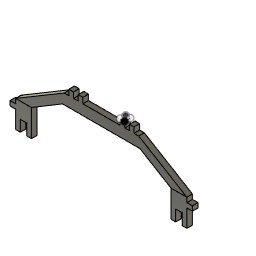
Test frame parts v2 (Autodesk Fusion 360 archive; units mm, degrees)
design "Test Carry Legs"
Autodesk Fusion 360 part; units mm, degrees
sketch "Sketch1" plane through (0, 0, 0) normal (0, 0, 1) x (1, 0, 0) in component "sidelegs"
  line L0 (-75, -45) -> (-92, -45)
  line L1 (-92, -45) -> (-92, -39)
  line L2 (-92, -39) -> (-75, -39)
  line L3 (-75, -39) -> (-75, -45)
  line L4 (75, -45) -> (92, -45)
  line L5 (92, -45) -> (92, -39)
  line L6 (92, -39) -> (75, -39)
  line L7 (75, -39) -> (75, -45)
  dimension "d7" = 17
  dimension "d8" = 6
  dimension "d9" = 17
  dimension "d10" = 6
  constraint horizontal L0
  constraint vertical L1
  constraint horizontal L2
  constraint vertical L3
  constraint horizontal L4
  constraint vertical L5
  constraint horizontal L6
  constraint vertical L7
  measures "d7" distance of L0.start L0.end
  measures "d8" distance of L0.start L2.end
  measures "d9" distance of L4.start L4.end
  measures "d10" distance of L4.start L6.end
extrude "Extrude1" add sketch "Sketch1" along normal blind 17 makes body 1 at (-80.6667, -45, 11.3333) makes body 2 at (86.3333, -39, 11.3333) in component "sidelegs"
sketch "Sketch2" plane through (0, -45, 0) normal (0, -1, 0) x (1, 0, 0) in component "sidelegs"
  line L0 (-92, 0) -> (-75, 0)
  line L1 (-75, 0) -> (-75, 17)
  line L2 (-75, 17) -> (-92, 17)
  line L3 (-92, 17) -> (-92, 0)
  line L4 (-75, 17) -> (-41.5705, 37.0865)
  line L5 (-75, 17) -> (-36, 17) construction
  line L6 (75, 17) -> (41.5705, 37.0865)
  line L7 (75, 17) -> (114, 17) construction
  line L8 (-41.5705, 37.0865) -> (41.5705, 37.0865)
  line L9 (92, 17) -> (40.2293, 48.107)
  line L10 (40.2293, 48.107) -> (-39.7707, 48.107)
  line L11 (-39.7707, 48.107) -> (-92, 17)
  line L12 (75, 17) -> (92, 17)
  line L13 (-75, 17) -> (-92, 17)
  dimension "d13" = 39
  dimension "d14" = 31
  dimension "d15" = 149
  dimension "d16" = 39
  dimension "d25" = 80
  constraint horizontal L5
  constraint coincident L1.end L2.start
  constraint horizontal L7
  constraint coincident L7 L9.start
  constraint parallel L6 L9
  constraint parallel L7 L10
  constraint coincident L2.end L3.start
  measures "d13" distance of L1.end L4.end
  measures "d14" angle of L4 L5
  measures "d15" angle of L6 L7
  measures "d16" distance of L6.start L6.end
  measures "d25" distance of L9.end L10.end
extrude "Extrude2" add sketch "Sketch2" against normal blind 6 separate body contours L2 L4 L6 L8 L9 L10 L11 L12 L13 makes body 3 in component "sidelegs"
sketch "Sketch3" plane through (0, 0, 0) normal (0, 0, -1) x (1, 0, 0) in component "sidelegs"
  line L0 (-92, 39) -> (-75, 39)
  line L1 (-75, 39) -> (-75, 45)
  line L2 (-75, 45) -> (-92, 45)
  line L3 (-92, 45) -> (-92, 39)
  line L4 (-92, 45) -> (-87, 45)
  line L5 (-87, 45) -> (-87, 39)
  line L6 (-87, 39) -> (-92, 39)
  line L7 (-92, 39) -> (-92, 45)
  line L8 (-75, 45) -> (-80, 45)
  line L9 (-80, 45) -> (-80, 39)
  line L10 (-80, 39) -> (-75, 39)
  line L11 (-75, 39) -> (-75, 45)
  constraint horizontal L4
  constraint vertical L5
  constraint horizontal L6
  constraint vertical L7
  constraint coincident L0 L5.end
  constraint coincident L2.end L3.start
  constraint horizontal L8
  constraint vertical L9
  constraint horizontal L10
  constraint vertical L11
  constraint coincident L0 L9.end
  constraint coincident L1.end L2.start
extrude "Extrude3" add sketch "Sketch3" along normal blind 12 contours L0 L2 L3 L4 L5 L6 L7 | L0 L1 L2 L8 L9 L10 L11 bodies 1 in component "sidelegs"
ref_plane "WorkPlane1" through (0, 0, 0) normal (1, 0, 0) x (0, 1, 0) in component "sidelegs"
sketch "Sketch4" plane through (0, 0, 0) normal (0, 0, -1) x (1, 0, 0) in component "sidelegs"
  line L0 (75, 45) -> (75, 39)
  line L1 (75, 39) -> (92, 39)
  line L2 (92, 39) -> (92, 45)
  line L3 (92, 45) -> (75, 45)
  line L4 (92, 39) -> (87, 39)
  line L5 (87, 39) -> (87, 45)
  line L6 (87, 45) -> (92, 45)
  line L7 (92, 45) -> (92, 39)
  line L8 (75, 39) -> (80, 39)
  line L9 (80, 39) -> (80, 45)
  line L10 (80, 45) -> (75, 45)
  line L11 (75, 45) -> (75, 39)
  constraint horizontal L4
  constraint vertical L5
  constraint horizontal L6
  constraint vertical L7
  constraint coincident L3 L5.end
  constraint coincident L1.end L2.start
  constraint horizontal L8
  constraint vertical L9
  constraint horizontal L10
  constraint vertical L11
  constraint coincident L3 L9.end
  constraint coincident L0.end L1.start
extrude "Extrude4" add sketch "Sketch4" along normal blind 12 contours L0 L1 L3 L8 L9 L10 L11 | L1 L2 L3 L4 L5 L6 L7 bodies 2 in component "sidelegs"
sketch "Sketch5" plane through (0, 0, 48.107) normal (0, 0, 1) x (-1, 0, 0) in component "sidelegs"
  line L0 (39.7707, 45) -> (-40.2293, 45)
  line L1 (-40.2293, 45) -> (-40.2293, 39)
  line L2 (-40.2293, 39) -> (39.7707, 39)
  line L3 (39.7707, 39) -> (39.7707, 45)
  line L4 (-40.2293, 45) -> (-35.2293, 45) construction
  line L5 (-35.2293, 45) -> (-35.2293, 39) construction
  line L6 (-35.2293, 39) -> (-40.2293, 39) construction
  line L7 (-40.2293, 39) -> (-40.2293, 45) construction
  line L8 (39.7707, 45) -> (34.7707, 45) construction
  line L9 (34.7707, 45) -> (34.7707, 39) construction
  line L10 (34.7707, 39) -> (39.7707, 39) construction
  line L11 (39.7707, 39) -> (39.7707, 45) construction
  line L12 (-35.2293, 45) -> (-30.2293, 45) construction
  line L13 (-30.2293, 45) -> (-30.2293, 39) construction
  line L14 (-30.2293, 39) -> (-35.2293, 39) construction
  line L15 (-35.2293, 39) -> (-35.2293, 45) construction
  line L16 (-30, 45) -> (-25, 45) construction
  line L17 (-25, 45) -> (-25, 39) construction
  line L18 (-25, 39) -> (-30, 39) construction
  line L19 (-30, 39) -> (-30, 45) construction
  line L20 (34.7707, 45) -> (29.7707, 45) construction
  line L21 (29.7707, 45) -> (29.7707, 39) construction
  line L22 (29.7707, 39) -> (34.7707, 39) construction
  line L23 (34.7707, 39) -> (34.7707, 45) construction
  line L24 (29.7707, 45) -> (24.7707, 45) construction
  line L25 (24.7707, 45) -> (24.7707, 39) construction
  line L26 (24.7707, 39) -> (29.7707, 39) construction
  line L27 (29.7707, 39) -> (29.7707, 45) construction
  line L28 (34.7707, 45) -> (29.7707, 45)
  line L29 (29.7707, 45) -> (29.7707, 39)
  line L30 (29.7707, 39) -> (34.7707, 39)
  line L31 (34.7707, 39) -> (34.7707, 45)
  line L32 (-35.2293, 45) -> (-30, 45)
  line L33 (-30, 45) -> (-30, 39)
  line L34 (-30, 39) -> (-35.2293, 39)
  line L35 (-35.2293, 39) -> (-35.2293, 45)
  line L36 (-25, 45) -> (-20, 45)
  line L37 (-20, 45) -> (-20, 39)
  line L38 (-20, 39) -> (-25, 39)
  line L39 (-25, 39) -> (-25, 45)
  line L40 (24.7707, 45) -> (19.7707, 45)
  line L41 (19.7707, 45) -> (19.7707, 39)
  line L42 (19.7707, 39) -> (24.7707, 39)
  line L43 (24.7707, 39) -> (24.7707, 45)
  dimension "d26" = 5
  dimension "d27" = 5
  dimension "d28" = 5
  dimension "d29" = 5
  dimension "d30" = 5
  dimension "d31" = 5
  dimension "d32" = 5
  constraint horizontal L4
  constraint vertical L5
  constraint horizontal L6
  constraint vertical L7
  constraint coincident L2 L5.end
  constraint coincident L0.end L1.start
  constraint horizontal L8
  constraint vertical L9
  constraint horizontal L10
  constraint vertical L11
  constraint coincident L2 L9.end
  constraint coincident L0.start L3.end
  constraint horizontal L12
  constraint vertical L13
  constraint horizontal L14
  constraint vertical L15
  constraint coincident L2 L13.end
  constraint horizontal L16
  constraint vertical L17
  constraint horizontal L18
  constraint vertical L19
  constraint coincident L0 L16.start
  constraint horizontal L20
  constraint vertical L21
  constraint horizontal L22
  constraint vertical L23
  constraint coincident L2 L21.end
  constraint horizontal L24
  constraint vertical L25
  constraint horizontal L26
  constraint vertical L27
  constraint coincident L2 L25.end
  constraint horizontal L28
  constraint vertical L29
  constraint horizontal L30
  constraint vertical L31
  constraint horizontal L32
  constraint vertical L33
  constraint horizontal L34
  constraint vertical L35
  constraint horizontal L36
  constraint vertical L37
  constraint horizontal L38
  constraint vertical L39
  constraint coincident L2 L37.end
  constraint horizontal L40
  constraint vertical L41
  constraint horizontal L42
  constraint vertical L43
  measures "d26" distance of L0.end L4.end
  measures "d27" distance of L0.start L8.end
  measures "d28" distance of L4.end L12.end
  measures "d29" distance of L16.start L16.end
  measures "d30" distance of L8.end L20.end
  measures "d31" distance of L20.end L24.end
  measures "d32" distance of L24.end L40.end
extrude "Extrude5" add sketch "Sketch5" along normal blind 6 contours L0 L2 L28 L29 L30 L31 | L0 L2 L40 L41 L42 L43 | L0 L2 L36 L37 L38 L39 | L0 L2 L32 L33 L34 L35 bodies 3 in component "sidelegs"
sketch "Sketch6" plane through (-92, 0, 0) normal (-1, 0, 0) x (0, -1, 0) in component "sidelegs"
  line L0 (45, -12) -> (45, 17)
  line L1 (45, 17) -> (39, 17)
  line L2 (39, 17) -> (39, -12)
  line L3 (39, -12) -> (45, -12)
  line L4 (45, 17) -> (45, 0) construction
  line L5 (39, 0) -> (39, 17) construction
  line L6 (39, 17) -> (45, 17) construction
  line L7 (45, 17) -> (45, 12) construction
  line L8 (45, 12) -> (39, 12) construction
  line L9 (39, 12) -> (39, 17) construction
  line L10 (39, 12) -> (45, 12)
  line L11 (45, 12) -> (45, 7)
  line L12 (45, 7) -> (39, 7)
  line L13 (39, 7) -> (39, 12)
  constraint coincident L0.end L1.start
  constraint coincident L0 L4.end
  constraint perpendicular L1 L4
  constraint coincident L2 L5.start
  constraint coincident L1.end L2.start
  constraint horizontal L6
  constraint vertical L7
  constraint horizontal L8
  constraint vertical L9
  constraint coincident L4 L7.end
  constraint horizontal L10
  constraint vertical L11
  constraint horizontal L12
  constraint vertical L13
  constraint coincident L4 L11.end
extrude "Extrude6" add sketch "Sketch6" along normal blind 6 contours L0 L2 L10 L11 L12 L13 bodies 1 in component "sidelegs"
sketch "Sketch7" plane through (92, 0, 0) normal (1, 0, 0) x (0, 1, 0) in component "sidelegs"
  line L0 (-39, -12) -> (-39, 17)
  line L1 (-39, 17) -> (-45, 17)
  line L2 (-45, 17) -> (-45, -12)
  line L3 (-45, -12) -> (-39, -12)
  line L4 (-45, 17) -> (-39, 17) construction
  line L5 (-39, 17) -> (-39, 12) construction
  line L6 (-39, 12) -> (-45, 12) construction
  line L7 (-45, 12) -> (-45, 17) construction
  line L8 (-45, 12) -> (-39, 12)
  line L9 (-39, 12) -> (-39, 7)
  line L10 (-39, 7) -> (-45, 7)
  line L11 (-45, 7) -> (-45, 12)
  constraint horizontal L4
  constraint vertical L5
  constraint horizontal L6
  constraint vertical L7
  constraint coincident L0 L5.end
  constraint coincident L1.end L2.start
  constraint horizontal L8
  constraint vertical L9
  constraint horizontal L10
  constraint vertical L11
  constraint coincident L0 L9.end
extrude "Extrude7" add sketch "Sketch7" along normal blind 6 contours L0 L2 L8 L9 L10 L11 bodies 2 in component "sidelegs"
sketch "Sketch8" plane through (0, 0, 54.107) normal (0, 0, 1) x (-1, 0, 0) in component "sidelegs"
  line L0 (-35.2293, 39) -> (-30, 39)
  line L1 (-30, 39) -> (-30, 45)
  line L2 (-30, 45) -> (-35.2293, 45)
  line L3 (-35.2293, 45) -> (-35.2293, 39)
  line L4 (-30, 42) -> (-30.229, 42) construction
  line L5 (-30.229, 42) -> (-30.229, 39) construction
  line L6 (-30.229, 42) -> (-30.229, 45) construction
  line L7 (-30.229, 45) -> (-30, 45) construction
  line L8 (-30, 45) -> (-30, 39) construction
  line L9 (-30, 39) -> (-30.229, 39) construction
  line L10 (-30.229, 39) -> (-30.229, 45) construction
  line L11 (-30, 45) -> (-30.229, 45)
  line L12 (-30.229, 45) -> (-30.229, 39)
  line L13 (-30.229, 39) -> (-30, 39)
  line L14 (-30, 39) -> (-30, 45)
  dimension "d39" = 0.229
  constraint midpoint L1 L4.start
  constraint perpendicular L1 L4
  constraint coincident L0 L5.end
  constraint perpendicular L0 L5
  constraint coincident L2 L6.end
  constraint perpendicular L2 L6
  constraint horizontal L7
  constraint vertical L8
  constraint horizontal L9
  constraint vertical L10
  constraint coincident L0.end L1.start
  constraint horizontal L11
  constraint vertical L12
  constraint horizontal L13
  constraint vertical L14
  measures "d39" distance of L4.start L4.end
extrude "Extrude8" cut sketch "Sketch8" against normal blind 6 contours L0 L1 L2 L11 L12 L13 L14 bodies 3 in component "sidelegs"
sketch "Sketch9" plane through (0, 0, 54.107) normal (0, 0, 1) x (-1, 0, 0) in component "sidelegs"
  line L0 (-25, 39) -> (-20, 39)
  line L1 (-20, 39) -> (-20, 45)
  line L2 (-20, 45) -> (-25, 45)
  line L3 (-25, 45) -> (-25, 39)
  line L4 (-25, 45) -> (-25.229, 45)
  line L5 (-25.229, 45) -> (-25.229, 39)
  line L6 (-25.229, 39) -> (-25, 39)
  line L7 (-20.229, 45) -> (-20.229, 39)
  dimension "d42" = 0.229
  dimension "d43" = 6
  dimension "d46" = 0.229
  constraint horizontal L4
  constraint vertical L5
  constraint horizontal L6
  constraint coincident L2.end L3.start
  constraint vertical L7
  constraint coincident L0 L7.end
  measures "d42" distance of L2.end L4.end
  measures "d43" distance of L2.end L0.start
  measures "d46" distance of L1.end L7.start
extrude "Extrude9" add sketch "Sketch9" against normal blind 6 contours L3 L4 L5 L6 bodies 3 in component "sidelegs"
extrude "Extrude10" cut sketch "Sketch9" against normal blind 6 contours L0 L1 L2 L7 bodies 3 in component "sidelegs"
component "sidelegs" placed x (1, 0, 0) y (0, 1, 0) z (0, 0, 1) at (0, 0, 0)

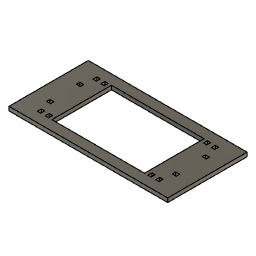
design "Test Base"
Autodesk Fusion 360 part; units mm, degrees
sketch "Sketch1" plane through (0, 0, 0) normal (0, 0, 1) x (1, 0, 0) in component "Base"
  line L0 (120, 60) -> (-120, 60)
  line L1 (-120, 60) -> (-120, -60)
  line L2 (-120, -60) -> (120, -60)
  line L3 (120, -60) -> (120, 60)
  line L4 (120, 60) -> (-120, -60) construction
  line L5 (-120, 60) -> (120, -60) construction
  line L6 (-70, 45) -> (70, 45)
  line L7 (70, 45) -> (70, -45)
  line L8 (70, -45) -> (-70, -45)
  line L9 (-70, -45) -> (-70, 45)
  line L10 (-70, 45) -> (70, -45) construction
  line L11 (70, 45) -> (-70, -45) construction
  dimension "d1" = 240
  dimension "d2" = 120
  dimension "d3" = 90
  dimension "d6" = 140
  constraint horizontal L0
  constraint perpendicular L0 L1
  constraint parallel L0 L2
  constraint parallel L1 L3
  constraint coincident L4 origin
  constraint coincident L5 origin
  constraint horizontal L6
  constraint perpendicular L6 L7
  constraint parallel L6 L8
  constraint parallel L7 L9
  constraint coincident L10 origin
  constraint coincident L11 origin
  measures "d1" distance of L1.end L2.end
  measures "d2" distance of L0.end L1.end
  measures "d3" distance of L6.end L7.end
  measures "d6" distance of L7 L9
extrude "Extrude1" add sketch "Sketch1" along normal blind 6 in component "Base"
sketch "Sketch2" plane through (0, 0, 6) normal (0, 0, 1) x (-1, 0, 0) in component "Base"
  line L0 (-70, 45) -> (70, 45)
  line L1 (70, 45) -> (70, -45)
  line L2 (70, -45) -> (-70, -45)
  line L3 (-70, -45) -> (-70, 45)
  line L4 (-120, 60) -> (-120, -60)
  line L5 (-120, -60) -> (120, -60)
  line L6 (120, -60) -> (120, 60)
  line L7 (120, 60) -> (-120, 60)
  line L8 (70, 45) -> (92, 45) construction
  line L9 (92, 45) -> (92, 39) construction
  line L10 (92, 39) -> (70, 39) construction
  line L11 (70, 39) -> (70, 45) construction
  line L12 (92, 39) -> (87, 39)
  line L13 (87, 39) -> (87, 45)
  line L14 (87, 45) -> (92, 45)
  line L15 (92, 45) -> (92, 39)
  line L16 (70, 39) -> (75, 39) construction
  line L17 (75, 45) -> (75, 39) construction
  line L18 (75, 39) -> (80, 39)
  line L19 (80, 39) -> (80, 45)
  line L20 (80, 45) -> (75, 45)
  line L21 (75, 45) -> (75, 39)
  dimension "d15" = 6
  constraint horizontal L8
  constraint vertical L9
  constraint horizontal L10
  constraint vertical L11
  constraint coincident L0.end L1.start
  constraint horizontal L12
  constraint vertical L13
  constraint horizontal L14
  constraint vertical L15
  constraint coincident L8 L13.end
  constraint coincident L10 L16.end
  constraint coincident L8 L17.start
  constraint perpendicular L10 L17
  constraint horizontal L18
  constraint vertical L19
  constraint horizontal L20
  constraint vertical L21
  constraint coincident L8 L19.end
  measures "d15" distance of L8 L12
extrude "Extrude2" cut sketch "Sketch2" against normal blind 6 contours L12 L13 L14 L15 | L18 L19 L20 L21 in component "Base"
ref_plane "WorkPlane1" through (0, 0, 0) normal (1, 0, 0) x (0, 1, 0) in component "Base"
mirror "Mirror1" about plane through (0, 0, 0) normal (1, 0, 0) of "Extrude2" in component "Base"
ref_plane "WorkPlane2" through (0, 0, 0) normal (0, 1, 0) x (0, 0, 1) in component "Base"
mirror "Mirror2" about plane through (0, 0, 0) normal (0, 1, 0) of "Extrude2", "Mirror1" in component "Base"
sketch "Sketch3" plane through (0, 0, 0) normal (0, 0, -1) x (1, 0, 0) in component "Base"
  line L0 (87, -45) -> (87, -39)
  line L1 (87, -39) -> (92, -39)
  line L2 (92, -39) -> (92, -45)
  line L3 (92, -45) -> (87, -45)
  line L4 (75, -39) -> (80, -39)
  line L5 (80, -39) -> (80, -45)
  line L6 (80, -45) -> (75, -45)
  line L7 (75, -45) -> (75, -39)
  line L8 (-87, -39) -> (-87, -45)
  line L9 (-87, -45) -> (-92, -45)
  line L10 (-92, -45) -> (-92, -39)
  line L11 (-92, -39) -> (-87, -39)
  line L12 (-80, -39) -> (-75, -39)
  line L13 (-75, -39) -> (-75, -45)
  line L14 (-75, -45) -> (-80, -45)
  line L15 (-80, -45) -> (-80, -39)
  line L16 (87, 39) -> (87, 45)
  line L17 (87, 45) -> (92, 45)
  line L18 (92, 45) -> (92, 39)
  line L19 (92, 39) -> (87, 39)
  line L20 (80, 39) -> (75, 39)
  line L21 (75, 39) -> (75, 45)
  line L22 (75, 45) -> (80, 45)
  line L23 (80, 45) -> (80, 39)
  line L24 (-87, 45) -> (-87, 39)
  line L25 (-87, 39) -> (-92, 39)
  line L26 (-92, 39) -> (-92, 45)
  line L27 (-92, 45) -> (-87, 45)
  line L28 (-75, 39) -> (-80, 39)
  line L29 (-80, 39) -> (-80, 45)
  line L30 (-80, 45) -> (-75, 45)
  line L31 (-75, 45) -> (-75, 39)
  line L32 (-70, 45) -> (70, 45)
  line L33 (70, 45) -> (70, -45)
  line L34 (70, -45) -> (-70, -45)
  line L35 (-70, -45) -> (-70, 45)
  line L36 (120, -60) -> (120, 60)
  line L37 (120, 60) -> (-120, 60)
  line L38 (-120, 60) -> (-120, -60)
  line L39 (-120, -60) -> (120, -60)
  line L40 (-120, 0) -> (-70, 0) construction
  line L41 (-87, -39) -> (-87, 39) construction
  line L42 (-87, 0) -> (-87, -20) construction
  line L43 (-87, 0) -> (-87, -20) construction
  line L44 (-87, 0) -> (-93, 0) construction
  line L45 (-87, 0) -> (-92, 0) construction
  line L46 (-92, 0) -> (-92, -20) construction
  line L47 (-92, -20) -> (-87, -20) construction
  line L48 (-87, -20) -> (-87, 0) construction
  line L49 (-87, 0) -> (-91.9449, 0) construction
  line L50 (-91.9449, 20) -> (-87, 20) construction
  line L51 (-87, 20) -> (-87, 0) construction
  line L52 (-87, 0) -> (-92, 0) construction
  line L53 (-92, 0) -> (-92, 20) construction
  line L54 (-92, 20) -> (-87, 20) construction
  line L55 (-87, 20) -> (-87, 0) construction
  line L56 (-92, -20) -> (-98, -20)
  line L57 (-98, -20) -> (-98, -25)
  line L58 (-98, -25) -> (-92, -25)
  line L59 (-92, -25) -> (-92, -20)
  line L60 (-92, 20) -> (-98, 20)
  line L61 (-98, 20) -> (-98, 25)
  line L62 (-98, 25) -> (-92, 25)
  line L63 (-92, 25) -> (-92, 20)
  dimension "d16" = 5
  dimension "d17" = 20
  dimension "d18" = 20
  constraint midpoint L38 L40.start
  constraint midpoint L35 L40.end
  constraint coincident L8.start L11.end
  constraint coincident L24.end L25.start
  constraint midpoint L41 L42.start
  constraint coincident L41 L42.end
  constraint perpendicular L40 L42
  constraint coincident L40 L44.end
  constraint perpendicular L41 L44
  constraint horizontal L45
  constraint vertical L46
  constraint horizontal L47
  constraint vertical L48
  constraint horizontal L49
  constraint horizontal L50
  constraint vertical L51
  constraint horizontal L52
  constraint vertical L53
  constraint horizontal L54
  constraint vertical L55
  constraint horizontal L56
  constraint vertical L57
  constraint horizontal L58
  constraint vertical L59
  constraint horizontal L60
  constraint vertical L61
  constraint horizontal L62
  constraint vertical L63
  measures "d16" distance of L42.start L45.end
  measures "d17" distance of L42.start L42.end
  measures "d18" distance of L42.start L50.end
extrude "Extrude3" cut sketch "Sketch3" against normal blind 11 contours L56 L57 L58 L59 | L60 L61 L62 L63 in component "Base"
mirror "Mirror3" about plane through (0, 0, 0) normal (1, 0, 0) of "Extrude3" in component "Base"
component "Base" placed x (1, 0, 0) y (0, 1, 0) z (0, 0, 1) at (0, 0, 0)

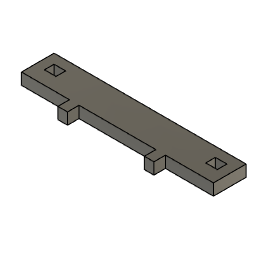
design "North/South Plank"
Autodesk Fusion 360 part; units mm, degrees
sketch "Sketch1" plane through (0, 0, 0) normal (0, 0, 1) x (1, 0, 0)
  line L0 (-45, 8.5) -> (45, 8.5)
  line L1 (45, 8.5) -> (45, -8.5)
  line L2 (45, -8.5) -> (-45, -8.5)
  line L3 (-45, -8.5) -> (-45, 8.5)
  line L4 (-45, 8.5) -> (45, -8.5) construction
  line L5 (45, 8.5) -> (-45, -8.5) construction
  dimension "d1" = 90
  dimension "d2" = 17
  constraint horizontal L0
  constraint perpendicular L0 L1
  constraint parallel L0 L2
  constraint parallel L1 L3
  constraint coincident L4 origin
  constraint coincident L5 origin
  measures "d1" distance of L1.end L2.end
  measures "d2" distance of L0.end L1.end
extrude "Extrude1" add sketch "Sketch1" along normal blind 6
sketch "Sketch2" plane through (0, 0, 6) normal (0, 0, 1) x (-1, 0, 0)
  line L0 (45, 8.5) -> (-45, 8.5)
  line L1 (-45, 8.5) -> (-45, -8.5)
  line L2 (-45, -8.5) -> (45, -8.5)
  line L3 (45, -8.5) -> (45, 8.5)
  line L4 (45, -8.5) -> (39, -8.5) construction
  line L5 (39, -8.5) -> (39, -3.5) construction
  line L6 (39, -3.5) -> (45, -3.5) construction
  line L7 (45, -3.5) -> (45, -8.5) construction
  line L8 (-45, -8.5) -> (-39, -8.5) construction
  line L9 (-39, -8.5) -> (-39, -3.5) construction
  line L10 (-39, -3.5) -> (-45, -3.5) construction
  line L11 (-45, -3.5) -> (-45, -8.5) construction
  line L12 (45, -3.5) -> (39, -3.5)
  line L13 (39, -3.5) -> (39, 1.5)
  line L14 (39, 1.5) -> (45, 1.5)
  line L15 (45, 1.5) -> (45, -3.5)
  line L16 (-45, -3.5) -> (-39, -3.5)
  line L17 (-39, -3.5) -> (-39, 1.5)
  line L18 (-39, 1.5) -> (-45, 1.5)
  line L19 (-45, 1.5) -> (-45, -3.5)
  dimension "d5" = 6
  dimension "d6" = 5
  dimension "d7" = 6
  dimension "d8" = 5
  dimension "d9" = 5
  dimension "d10" = 5
  constraint horizontal L4
  constraint vertical L5
  constraint horizontal L6
  constraint vertical L7
  constraint coincident L2.end L3.start
  constraint horizontal L8
  constraint vertical L9
  constraint horizontal L10
  constraint vertical L11
  constraint coincident L1.end L2.start
  constraint horizontal L12
  constraint vertical L13
  constraint horizontal L14
  constraint vertical L15
  constraint horizontal L16
  constraint vertical L17
  constraint horizontal L18
  constraint vertical L19
  measures "d5" distance of L2.end L4.end
  measures "d6" distance of L2.end L6.end
  measures "d7" distance of L1.end L8.end
  measures "d8" distance of L1.end L10.end
  measures "d9" distance of L6.end L14.end
  measures "d10" distance of L10.end L18.end
extrude "Extrude2" cut sketch "Sketch2" against normal blind 9 contours L3 L12 L13 L14 L15 | L1 L16 L17 L18 L19
sketch "Sketch3" plane through (0, -8.5, 0) normal (0, -1, 0) x (1, 0, 0)
  line L0 (-45, 0) -> (45, 0)
  line L1 (45, 0) -> (45, 6)
  line L2 (45, 6) -> (-45, 6)
  line L3 (-45, 6) -> (-45, 0)
  line L4 (0, 6) -> (39, 6) construction
  line L5 (39, 0) -> (39, 6) construction
  line L6 (0, 6) -> (-39, 6) construction
  line L7 (-39, 6) -> (-39, 0) construction
  line L8 (0, 6) -> (0, 0)
  line L9 (0, 2.5249) -> (-20, 2.5249) construction
  line L10 (-20, 2.5249) -> (-20, 0) construction
  line L11 (0, 2.5249) -> (20, 2.5249) construction
  line L12 (-20, 0) -> (-25, 0)
  line L13 (-25, 0) -> (-25, 6)
  line L14 (-25, 6) -> (-20, 6)
  line L15 (-20, 6) -> (-20, 0)
  line L16 (20, 0) -> (25, 0)
  line L17 (25, 0) -> (25, 6)
  line L18 (25, 6) -> (20, 6)
  line L19 (20, 6) -> (20, 0)
  constraint midpoint L2 L4.start
  constraint coincident L2 L4.end
  constraint parallel L2 L4
  constraint coincident L0 L5.start
  constraint perpendicular L4 L5
  constraint coincident L2 L6.end
  constraint perpendicular L5 L6
  constraint coincident L0 L7.end
  constraint perpendicular L0 L7
  constraint coincident L8.end origin
  constraint coincident L8 L9.start
  constraint perpendicular L8 L9
  constraint coincident L0 L10.end
  constraint perpendicular L0 L10
  constraint perpendicular L8 L11
  constraint horizontal L12
  constraint vertical L13
  constraint horizontal L14
  constraint vertical L15
  constraint coincident L6 L13.end
  constraint horizontal L16
  constraint vertical L17
  constraint horizontal L18
  constraint vertical L19
  constraint coincident L4 L17.end
  constraint coincident L0 L16.start
extrude "Extrude3" add sketch "Sketch3" along normal blind 6 contours L0 L2 L12 L13 L14 L15 | L0 L2 L16 L17 L18 L19
sketch "Sketch4" plane through (-45, 0, 0) normal (-1, 0, 0) x (0, -1, 0)
  line L0 (-3.5, 0) -> (-3.5, 6)
  line L1 (-3.5, 6) -> (-8.5, 6)
  line L2 (-8.5, 6) -> (-8.5, 0)
  line L3 (-8.5, 0) -> (-3.5, 0)
  line L4 (-8.5, 6) -> (8.5, 6)
  line L5 (8.5, 6) -> (8.5, 0)
  line L6 (8.5, 0) -> (-8.5, 0)
  line L7 (-8.5, 0) -> (-8.5, 6)
  dimension "d15" = 17
  dimension "d16" = 6
  constraint horizontal L4
  constraint vertical L5
  constraint horizontal L6
  constraint vertical L7
  constraint coincident L1.end L2.start
  measures "d15" distance of L1.end L4.end
  measures "d16" distance of L1.end L2.end
extrude "Extrude4" add sketch "Sketch4" along normal blind 5
sketch "Sketch5" plane through (45, 0, 0) normal (1, 0, 0) x (0, 1, 0)
  line L0 (-1.5, 0) -> (-1.5, 6)
  line L1 (-1.5, 6) -> (-8.5, 6)
  line L2 (-8.5, 6) -> (-8.5, 0)
  line L3 (-8.5, 0) -> (-1.5, 0)
  line L4 (-8.5, 6) -> (8.5, 6)
  line L5 (8.5, 6) -> (8.5, 0)
  line L6 (8.5, 0) -> (-8.5, 0)
  line L7 (-8.5, 0) -> (-8.5, 6)
  dimension "d19" = 17
  constraint horizontal L4
  constraint vertical L5
  constraint horizontal L6
  constraint vertical L7
  constraint coincident L1.end L2.start
  measures "d19" distance of L1.end L4.end
extrude "Extrude5" add sketch "Sketch5" along normal blind 5

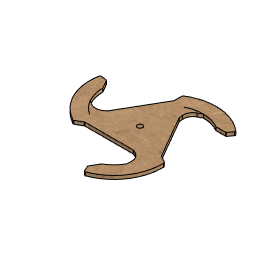
design "Hook Wheel 1/3 Size"
Autodesk Fusion 360 part; units mm, degrees
sketch "Sketch1" plane through (0, 0, 0) normal (0, 0, 1) x (1, 0, 0)
  line L0 (0, 0) -> (140, 0) construction
  line L1 (-106.2269, -44.0096) -> (-15, 114)
  line L2 (15, 114) -> (106.2269, -44.0096)
  line L3 (91.2269, -69.9904) -> (-91.2269, -69.9904)
  line L4 (-15, 140) -> (15, 140)
  line L5 (15, 140) -> (15, 114)
  line L6 (-15, 114) -> (-15, 140)
  line L7 (15, 140) -> (14.2708, 139.2708) construction
  line L8 (-128.7436, -57.0096) -> (-106.2269, -44.0096)
  line L9 (-113.7436, -82.9904) -> (-128.7436, -57.0096)
  line L10 (-91.2269, -69.9904) -> (-113.7436, -82.9904)
  line L11 (113.7436, -82.9904) -> (91.2269, -69.9904)
  line L12 (128.7436, -57.0096) -> (113.7436, -82.9904)
  line L13 (106.2269, -44.0096) -> (128.7436, -57.0096)
  dimension "d5" = 30
  dimension "d6" = 26
  dimension "d7" = 26
  dimension "d8" = 26
  dimension "d9" = 30
  dimension "d10" = 26
  dimension "d11" = 30
  dimension "d12" = 26
  dimension "d13" = 26
  constraint horizontal L0
  constraint coincident L0.start origin
  constraint horizontal L3
  constraint horizontal L4
  constraint perpendicular L4 L5
  constraint parallel L5 L6
  measures "d5" distance of L4.start L4.end
  measures "d6" distance of L4.end L2.start
  measures "d7" distance of L4.start L1.end
  measures "d8" distance of L12.start L2.end
  measures "d9" distance of L11.start L12.start
  measures "d10" distance of L11.start L3.start
  measures "d11" distance of L8.start L9.start
  measures "d12" distance of L8.start L1.start
  measures "d13" distance of L9.start L3.end
extrude "Extrude1" add sketch "Sketch1" along normal blind 10 makes body 1
fillet "Fillet1" radius 3 12 edges at (-113.7436, -82.9904, 5) (-91.2269, -69.9904, 5) (91.2269, -69.9904, 5) (113.7436, -82.9904, 5) (-128.7436, -57.0096, 5) (-106.2269, -44.0096, 5) (-15, 114, 5) (-15, 140, 5) (15, 140, 5) (15, 114, 5) (106.2269, -44.0096, 5) (128.7436, -57.0096, 5) on bodies 1
sketch "Sketch2" plane through (0, 0, 0) normal (0, 0, 1) x (1, 0, 0)
  line L0 (240.6616, 203.5291) -> (270, 203.5291)
  line L1 (270, 203.5291) -> (282.3476, 220.2232)
  line L2 (139.3384, 203.5291) -> (115.9466, 203.5291)
  line L3 (115.9466, 203.5291) -> (115.9466, 233.8111)
  arc A0 (240.6616, 203.5291) -> (139.3384, 203.5291) centre (190, 115) ccw
  arc A1 (282.3476, 220.2232) -> (115.9466, 233.8111) centre (190, 115) ccw
  dimension "d18" = 280
  constraint horizontal L0
  constraint parallel L0 L2
  constraint perpendicular L2 L3
  constraint concentric A0 A1
  measures "d18" diameter of A1
extrude "Extrude2" add sketch "Sketch2" along normal blind 10 separate body makes body 2
fillet "Fillet2" radius 3 2 edges at (115.9466, 203.5291, 5) (282.3476, 220.2232, 5) on bodies 2
sketch "Sketch3" plane through (0, 0, 10) normal (0, 0, 1) x (-1, 0, 0)
  arc A0 (-127.2436, 59.6077) -> (-126.1455, 55.5096) centre (-124.6455, 58.1077) ccw
  line L0 (-126.1455, 55.5096) -> (-106.9231, 44.4115)
  arc A1 (-105.825, 43.3134) -> (-106.9231, 44.4115) centre (-108.4231, 41.8134) ccw
  line L1 (-105.825, 43.3134) -> (-15.4019, -113.3038)
  arc A2 (-15, -114.8038) -> (-15.4019, -113.3038) centre (-18, -114.8038) ccw
  line L2 (-15, -114.8038) -> (-15, -137)
  arc A3 (-15, -137) -> (-12, -140) centre (-12, -137) ccw
  line L3 (-12, -140) -> (12, -140)
  arc A4 (12, -140) -> (15, -137) centre (12, -137) ccw
  line L4 (15, -137) -> (15, -114.8038)
  arc A5 (15.4019, -113.3038) -> (15, -114.8038) centre (18, -114.8038) ccw
  line L5 (15.4019, -113.3038) -> (105.825, 43.3134)
  arc A6 (106.9231, 44.4115) -> (105.825, 43.3134) centre (108.4231, 41.8134) ccw
  line L6 (106.9231, 44.4115) -> (126.1455, 55.5096)
  arc A7 (126.1455, 55.5096) -> (127.2436, 59.6077) centre (124.6455, 58.1077) ccw
  line L7 (127.2436, 59.6077) -> (115.2436, 80.3923)
  arc A8 (115.2436, 80.3923) -> (111.1455, 81.4904) centre (112.6455, 78.8923) ccw
  line L8 (111.1455, 81.4904) -> (91.923, 70.3923)
  arc A9 (90.423, 69.9904) -> (91.923, 70.3923) centre (90.423, 72.9904) ccw
  line L9 (90.423, 69.9904) -> (-90.423, 69.9904)
  arc A10 (-91.923, 70.3923) -> (-90.423, 69.9904) centre (-90.423, 72.9904) ccw
  line L10 (-91.923, 70.3923) -> (-111.1455, 81.4904)
  arc A11 (-111.1455, 81.4904) -> (-115.2436, 80.3923) centre (-112.6455, 78.8923) ccw
  line L11 (-115.2436, 80.3923) -> (-127.2436, 59.6077)
move_body "Move1" bodies 2 to x (1, 0, 0) y (0, 1, 0) z (0, 0, 1) at (0, -85, 0)
fillet "Fillet3" radius 1 2 edges at (240.6616, 118.5291, 5) (270, 118.5291, 5) on bodies 2
pattern_circular "C-Pattern1" count 3 over 360 about axis through (0, 0, 1.75) along (0, 0, 1) of bodies 2 makes body 3 at (-240.4651, 159.4049, 0) makes body 4 at (-17.8162, -287.9514, 0)
move_body "Move2" bodies 2 to x (1, 0, 0) y (0, 1, 0) z (0, 0, 1) at (-130, -10, 0)
move_body "Move3" bodies 4 to x (1, 0, 0) y (0, 1, 0) z (0, 0, 1) at (56.5, 116.5, 0)
move_body "Move4" bodies 2 to x (1, 0, 0) y (0, 1, 0) z (0, 0, 1) at (0.9, 0.8, 0)
move_body "Move5" bodies 3 to x (1, 0, 0) y (0, 1, 0) z (0, 0, 1) at (72.6, -107.2, 0)
move_body "Move6" bodies 2 to x (1, 0, 0) y (0, 1, 0) z (0, 0, 1) at (-0.09, -0.1, 0)
combine "Combine1" operation add target body 3 tool bodies 1
combine "Combine2" operation add target body 4 tool bodies 3
combine "Combine3" operation add target body 2 tool bodies 4
sketch "Sketch5" plane through (0, 0, 10) normal (0, 0, 1) x (-1, 0, 0)
  circle A0 centre (0, 0) radius 7.5
  dimension "d40" = 15
  constraint coincident A0.centre origin
  measures "d40" diameter of A0
extrude "Extrude7" cut sketch "Sketch5" against normal blind 10 bodies 2
sketch "Sketch1 (2)" plane through (0, 0, 10) normal (0, 0, 1) x (-1, 0, 0) in component "Component"
  circle A0 centre (0, 0) radius 7.5
  arc A1 (-111.2424, -109.3599) -> (-15.972, -112.3164) centre (-60.81, -20.7) ccw
  arc A2 (-111.2424, -109.3599) -> (-111.7368, -109.2291) centre (-111.7368, -110.2291) ccw
  line L0 (-111.7368, -109.2291) -> (-140.3058, -109.2291)
  arc A3 (-140.3058, -109.2291) -> (-141.1098, -109.6345) centre (-140.3058, -110.2291) ccw
  line L1 (-141.1098, -109.6345) -> (-151.5001, -123.6823)
  arc A4 (-151.5001, -123.6823) -> (-151.0213, -127.7604) centre (-149.0882, -125.4663) ccw
  arc A5 (-151.0213, -127.7604) -> (12.5301, -139.9528) centre (-60.81, -20.7) ccw
  arc A6 (12.5301, -139.9528) -> (15, -137) centre (12, -137) ccw
  line L2 (15, -137) -> (15, -114.8038)
  arc A7 (15.4019, -113.3038) -> (15, -114.8038) centre (18, -114.8038) ccw
  line L3 (15.4019, -113.3038) -> (105.2553, 42.3268)
  arc A8 (150.3787, -41.6906) -> (105.2553, 42.3268) centre (48.3808, -42.3448) ccw
  arc A9 (150.3787, -41.6906) -> (150.5126, -42.1842) centre (151.3786, -41.6842) ccw
  line L4 (150.5126, -42.1842) -> (164.7971, -66.9257)
  arc A10 (164.7971, -66.9257) -> (165.5502, -67.4193) centre (165.6632, -66.4257) ccw
  line L5 (165.5502, -67.4193) -> (182.9111, -69.3936)
  arc A11 (182.9111, -69.3936) -> (186.2034, -66.9399) centre (183.2501, -66.4128) ccw
  arc A12 (186.2034, -66.9399) -> (114.9458, 80.8181) centre (48.3808, -42.3448) ccw
  arc A13 (114.9458, 80.8181) -> (111.1455, 81.4904) centre (112.6455, 78.8923) ccw
  line L6 (111.1455, 81.4904) -> (91.923, 70.3923)
  arc A14 (90.423, 69.9904) -> (91.923, 70.3923) centre (90.423, 72.9904) ccw
  line L7 (90.423, 69.9904) -> (-89.244, 69.9904)
  arc A15 (-39.0463, 151.0505) -> (-89.244, 69.9904) centre (12.5192, 63.0448) ccw
  arc A16 (-39.0463, 151.0505) -> (-38.6858, 151.4133) centre (-39.5518, 151.9133) ccw
  line L8 (-38.6858, 151.4133) -> (-24.4013, 176.1548)
  arc A17 (-24.4013, 176.1548) -> (-24.3504, 177.0537) centre (-25.2673, 176.6548) ccw
  line L9 (-24.3504, 177.0537) -> (-31.321, 193.0759)
  arc A18 (-31.321, 193.0759) -> (-35.0922, 194.7003) centre (-34.0719, 191.8791) ccw
  arc A19 (-35.0922, 194.7003) -> (-127.4287, 59.2274) centre (12.5192, 63.0448) ccw
  arc A20 (-127.4287, 59.2274) -> (-126.1455, 55.5096) centre (-124.6455, 58.1077) ccw
  line L10 (-126.1455, 55.5096) -> (-106.9231, 44.4115)
  arc A21 (-105.825, 43.3134) -> (-106.9231, 44.4115) centre (-108.4231, 41.8134) ccw
  line L11 (-105.825, 43.3134) -> (-15.972, -112.3164)
  line L12 (-75.318, 114.8967) -> (-77, 82)
  line L13 (-77, 82) -> (-50.2742, 69.9904)
  constraint coincident A15 L12.start
  constraint coincident L7 L13.end
extrude "Extrude1'" add sketch "Sketch1 (2)" against normal blind 6 separate body contours L7 A15 L12 L13 makes body 5 in component "Component"
fillet "Fillet1'" radius 28 1 edges at (77, -82, 7) on bodies 5 in component "Component"
extrude "Extrude2'" add sketch "Sketch1 (2)" against normal blind 6 separate body contours A1 A2 L0 A3 L1 A4 A5 A6 L2 A7 L3 A8 A9 L4 A10 L5 A11 A12 A13 L6 A14 L7 A15 A16 L8 A17 L9 A18 A19 A20 L10 A21 L11 makes body 6 in component "Component"
pattern_circular "C-Pattern1'" count 3 over 360 about axis through (0, 0, 1.75) along (0, 0, 1) of bodies 5 makes body 7 at (26.3012, 110.0606, 10) makes body 8 at (-108.4659, -32.2528, 10) in component "Component"
extrude "Extrude3" add 3 faces at (-108.4659, -32.2528, 4) (82.1647, -77.8078, 4) (26.3012, 110.0606, 4) along direction (0, 0, -1) blind 4 on bodies 5 7 8 bodies 5 8 6 7 in component "Component"
combine "Combine4" operation add target body 2 tool bodies 5
scale "Scale1" factor 0.333 about (0, 0, 10) bodies 2
component "Component" placed x (1, 0, 0) y (0, 1, 0) z (0, 0, 1) at (0, 0, 0)

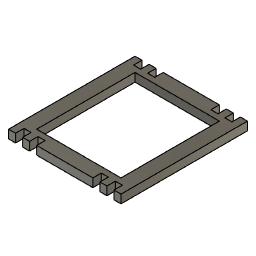
design "Carrier Top Piece"
Autodesk Fusion 360 part; units mm, degrees
sketch "Sketch1" plane through (0, 0, 0) normal (0, 0, 1) x (1, 0, 0)
  line L0 (40, 45) -> (-40, 45)
  line L1 (-40, 45) -> (-40, -45)
  line L2 (-40, -45) -> (40, -45)
  line L3 (40, -45) -> (40, 45)
  line L4 (40, 45) -> (-40, -45) construction
  line L5 (-40, 45) -> (40, -45) construction
  line L6 (30, 35) -> (-30, 35)
  line L7 (-30, 35) -> (-30, -35)
  line L8 (-30, -35) -> (30, -35)
  line L9 (30, -35) -> (30, 35)
  line L10 (30, 35) -> (-30, -35) construction
  line L11 (-30, 35) -> (30, -35) construction
  dimension "d1" = 80
  dimension "d2" = 90
  dimension "d3" = 60
  dimension "d6" = 10
  constraint horizontal L0
  constraint perpendicular L0 L1
  constraint parallel L0 L2
  constraint parallel L1 L3
  constraint coincident L4 origin
  constraint coincident L5 origin
  constraint horizontal L6
  constraint perpendicular L6 L7
  constraint parallel L6 L8
  constraint parallel L7 L9
  constraint coincident L10 origin
  constraint coincident L11 origin
  measures "d1" distance of L1.end L2.end
  measures "d2" distance of L0.end L1.end
  measures "d3" distance of L7.end L8.end
  measures "d6" distance of L0 L6
extrude "Extrude1" add sketch "Sketch1" along normal blind 6
sketch "Sketch2" plane through (0, 0, 6) normal (0, 0, 1) x (-1, 0, 0)
  line L0 (-30, -35) -> (-30, 35)
  line L1 (-30, 35) -> (30, 35)
  line L2 (30, 35) -> (30, -35)
  line L3 (30, -35) -> (-30, -35)
  line L4 (-40, 45) -> (-40, -45)
  line L5 (-40, -45) -> (40, -45)
  line L6 (40, -45) -> (40, 45)
  line L7 (40, 45) -> (-40, 45)
  line L8 (-40, 45) -> (-35, 45) construction
  line L9 (-35, 45) -> (-35, 39) construction
  line L10 (-35, 39) -> (-40, 39) construction
  line L11 (-40, 39) -> (-40, 45) construction
  line L12 (-35, 45) -> (-30, 45) construction
  line L13 (-30, 45) -> (-30, 39) construction
  line L14 (-30, 39) -> (-35, 39) construction
  line L15 (-35, 39) -> (-35, 45) construction
  line L16 (-30, 45) -> (-25, 45) construction
  line L17 (-25, 45) -> (-25, 39) construction
  line L18 (-25, 39) -> (-30, 39) construction
  line L19 (-30, 39) -> (-30, 45) construction
  line L20 (-25, 45) -> (-20, 45) construction
  line L21 (-20, 45) -> (-20, 39) construction
  line L22 (-20, 39) -> (-25, 39) construction
  line L23 (-25, 39) -> (-25, 45) construction
  line L24 (-30, 39) -> (-35, 39)
  line L25 (-35, 39) -> (-35, 45)
  line L26 (-35, 45) -> (-30, 45)
  line L27 (-30, 45) -> (-30, 39)
  line L28 (-20, 39) -> (-25, 39)
  line L29 (-25, 39) -> (-25, 45)
  line L30 (-25, 45) -> (-20, 45)
  line L31 (-20, 45) -> (-20, 39)
  line L32 (40, 45) -> (35, 45) construction
  line L33 (35, 45) -> (35, 39) construction
  line L34 (35, 39) -> (40, 39) construction
  line L35 (40, 39) -> (40, 45) construction
  line L36 (35, 39) -> (30, 39)
  line L37 (30, 39) -> (30, 45)
  line L38 (30, 45) -> (35, 45)
  line L39 (35, 45) -> (35, 39)
  line L40 (30, 39) -> (25, 39) construction
  line L41 (25, 39) -> (25, 45) construction
  line L42 (25, 45) -> (30, 45) construction
  line L43 (30, 45) -> (30, 39) construction
  line L44 (25, 39) -> (20, 39)
  line L45 (20, 39) -> (20, 45)
  line L46 (20, 45) -> (25, 45)
  line L47 (25, 45) -> (25, 39)
  constraint horizontal L8
  constraint vertical L9
  constraint horizontal L10
  constraint vertical L11
  constraint coincident L4.start L7.end
  constraint horizontal L12
  constraint vertical L13
  constraint horizontal L14
  constraint vertical L15
  constraint horizontal L16
  constraint vertical L17
  constraint horizontal L18
  constraint vertical L19
  constraint horizontal L20
  constraint vertical L21
  constraint horizontal L22
  constraint vertical L23
  constraint horizontal L24
  constraint vertical L25
  constraint horizontal L26
  constraint vertical L27
  constraint horizontal L28
  constraint vertical L29
  constraint horizontal L30
  constraint vertical L31
  constraint horizontal L32
  constraint vertical L33
  constraint horizontal L34
  constraint vertical L35
  constraint coincident L6.end L7.start
  constraint horizontal L36
  constraint vertical L37
  constraint horizontal L38
  constraint vertical L39
  constraint coincident L7 L37.end
  constraint horizontal L40
  constraint vertical L41
  constraint horizontal L42
  constraint vertical L43
  constraint coincident L7 L41.end
  constraint horizontal L44
  constraint vertical L45
  constraint horizontal L46
  constraint vertical L47
  constraint coincident L7 L45.end
extrude "Extrude2" cut sketch "Sketch2" against normal blind 6 contours L7 L24 L25 L26 L27 | L7 L28 L29 L30 L31
ref_plane "WorkPlane1" through (0, 0, 0) normal (0, 1, 0) x (0, 0, 1)
ref_plane "WorkPlane2" through (0, 0, 0) normal (1, 0, 0) x (0, 1, 0)
extrude "Extrude3" cut sketch "Sketch2" against normal blind 6 contours L7 L24 L25 L26 L27 | L7 L28 L29 L30 L31 | L7 L36 L37 L38 L39 | L7 L44 L45 L46 L47
mirror "Mirror3" about plane through (0, 0, 0) normal (0, 1, 0) of "Extrude3"
